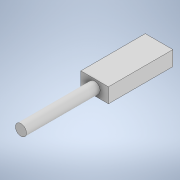
# Autodesk Inventor part: USBCable
Saved by Autodesk Inventor 2020 (Build 240168000, 168)
## iProperties
Created: 2019-12-18
Part Number: USBCable
Material: Generic
Document SubType Name: Modeling
Designer: nicoc
Density: 1 g/cm^3
Appearance: Default
Author: nicoc
Autodesk Inventor part; units mm, degrees
ref_plane "YZ Plane" through (0, 0, 0) normal (1, 0, 0) x (0, 1, 0)
ref_plane "XZ Plane" through (0, 0, 0) normal (0, 1, 0) x (-1, 0, 0)
ref_plane "XY Plane" through (0, 0, 0) normal (0, 0, 1) x (1, 0, 0)
sketch "Sketch1" plane through (0, 0, 0) normal (0, 1, 0) x (-1, 0, 0)
  line L0 (0, 0) -> (15, 0)
  line L1 (15, 0) -> (15, -35)
  line L2 (15, -35) -> (0, -35)
  line L3 (0, -35) -> (0, 0)
  dimension "d0" = 35
  dimension "d1" = 15
  constraints: 8 end point, 2 parallel, 1 horizontal, 1 perpendicular
  measures "d0" distance between parallel lines of L2 L0
  measures "d1" distance between parallel lines of L1 L3
extrude "Extrusion1" add sketch "Sketch1" along normal blind 8
sketch "Sketch2" plane through (-15, 0, 0) normal (0, 0, 1) x (1, 0, 0)
  circle A0 centre (7.5, 4) radius 3
  line L0 (15, 0) -> (15, 8) projected
  line L1 (0, 0) -> (15, 0) projected
  dimension "d4" = 7.5
  dimension "d5" = 4
  dimension "d6" = 6
  constraints: 1 centre point
  measures "d4" distance from line of A0.centre L0
  measures "d5" distance from line of A0.centre L1
  measures "d6" diameter of A0
extrude "Extrusion2" add sketch "Sketch2" along normal blind 40
body "Solid1"
